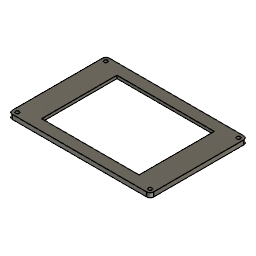
Lid V2 (Gasket) (Autodesk Fusion 360 design; units mm, degrees)
part number: 2026-01-29-14-58-12-979
Autodesk Fusion 360 part; units mm, degrees
sketch "Sketch2" plane through (0, 0, 0) normal (0, 0, 1) x (1, 0, 0)
  line L0 (-46, 50) -> (106, 50)
  line L1 (110, 46) -> (110, -56)
  line L2 (106, -60) -> (-46, -60)
  line L3 (-50, -56) -> (-50, 46)
  circle A0 centre (-45, 45) radius 2
  line L4 (30, -60) -> (30, 50) construction
  line L5 (-50, -5) -> (110, -5) construction
  arc A1 (-46, 50) -> (-50, 46) centre (-46, 46) ccw
  circle A2 centre (105, 45) radius 2
  arc A3 (110, 46) -> (106, 50) centre (106, 46) ccw
  circle A4 centre (105, -55) radius 2
  arc A5 (106, -60) -> (110, -56) centre (106, -56) ccw
  circle A6 centre (-45, -55) radius 2
  arc A7 (-50, -56) -> (-46, -60) centre (-46, -56) ccw
  point P0 (-50, 50)
  point P1 (110, 50)
  dimension "d3" = 4
  dimension "d4" = 5
  dimension "d5" = 5
  dimension "d6" = 4
  dimension "d63" = 160
  dimension "d64" = 110
  constraint horizontal L0
  constraint vertical L1
  constraint horizontal L2
  constraint vertical L3
  constraint coincident L0 L4.end
  constraint coincident L3 L5.start
  constraint coincident P0 L0
  constraint coincident P0 L3
  constraint tangent L0 A1
  constraint tangent L3 A1
  constraint symmetric P0 L4 P1
  constraint symmetric A0 L4 A2
  constraint symmetric L4 L0.start L0.end
  constraint symmetric L4 L3.end L1.start
  constraint symmetric L4 A1 A3
  constraint coincident L1 L5.end
  constraint symmetric A0 L5 A6
  constraint symmetric L5 L0.start L2.end
  constraint symmetric L5 L3.end L3.start
  constraint symmetric L5 A1 A7
  constraint symmetric L5 L1.start L1.end
  constraint symmetric L5 L0.end L2.start
  constraint symmetric L5 A2 A4
  constraint symmetric L5 A3 A5
  constraint coincident L2 L4.start
  measures "d3" diameter of A0
  measures "d4" distance of L0 A0.centre
  measures "d5" distance of L3 A0.centre
  measures "d6" radius of A1
  measures "d63" distance of L1 L3
  measures "d64" distance of L0 L2
extrude "Extrude1" add sketch "Sketch2" along normal blind 5
sketch "Sketch3" plane through (0, 0, 0) normal (0, 0, -1) x (1, 0, 0)
  circle A0 centre (105, 55) radius 2
  circle A1 centre (-45, 55) radius 2
  circle A2 centre (-45, -45) radius 2
  circle A3 centre (105, -45) radius 2
  arc A4 (-50, -46) -> (-46, -50) centre (-46, -46) ccw
  line L0 (-46, -50) -> (106, -50)
  arc A5 (106, -50) -> (110, -46) centre (106, -46) ccw
  line L1 (110, -46) -> (110, 56)
  arc A6 (110, 56) -> (106, 60) centre (106, 56) ccw
  line L2 (106, 60) -> (-46, 60)
  arc A7 (-46, 60) -> (-50, 56) centre (-46, 56) ccw
  line L3 (-50, 56) -> (-50, -46)
  line L4 (30, 60) -> (30, -50) construction
  line L5 (110, 5) -> (-50, 5) construction
  line L6 (101.7902, -41.7902) -> (-41.7901, -41.7902) construction
  line L7 (-41.7901, -41.7902) -> (-41.7901, 51.7901) construction
  line L8 (-41.7901, 51.7901) -> (101.7902, 51.7901) construction
  line L9 (101.7902, 51.7901) -> (101.7902, -41.7902) construction
  line L10 (101.7902, -41.7902) -> (-41.7901, 51.7901) construction
  line L11 (-41.7901, -41.7902) -> (101.7902, 51.7901) construction
  line L12 (95.2151, -42.8152) -> (-35.2152, -42.8152)
  line L13 (-42.8152, -35.2152) -> (-42.8152, 45.2151)
  line L14 (-35.2151, 52.8151) -> (95.2151, 52.8151)
  line L15 (102.8152, 45.2151) -> (102.8152, -35.2152)
  line L16 (88.9278, -33.6958) -> (-42.8152, 52.8151) construction
  line L17 (-37.4412, -35.28) -> (85.6746, 38.2522) construction
  line L18 (-40.7652, -35.2152) -> (-40.7652, 45.2152)
  line L19 (-35.2152, 50.7652) -> (95.2152, 50.7652)
  line L20 (100.7652, 45.2152) -> (100.7652, -35.2152)
  line L21 (98.2241, -39.1218) -> (-40.7652, 50.7652) construction
  line L22 (-34.7613, -32.5014) -> (82.9436, 35.6581) construction
  arc A8 (-35.2152, 50.7652) -> (-40.7652, 45.2152) centre (-35.2152, 45.2152) ccw
  arc A9 (-35.2151, 52.8151) -> (-42.8152, 45.2151) centre (-35.2152, 45.2151) ccw
  arc A10 (100.7652, 45.2152) -> (95.2152, 50.7652) centre (95.2152, 45.2152) ccw
  arc A11 (102.8152, 45.2151) -> (95.2151, 52.8151) centre (95.2152, 45.2151) ccw
  arc A12 (-40.7652, -35.2152) -> (-35.2152, -40.7652) centre (-35.2152, -35.2152) ccw
  arc A13 (-42.8152, -35.2152) -> (-35.2152, -42.8152) centre (-35.2152, -35.2152) ccw
  arc A14 (95.2152, -40.7652) -> (100.7652, -35.2152) centre (95.2152, -35.2152) ccw
  arc A15 (95.2151, -42.8152) -> (102.8151, -35.2152) centre (95.2151, -35.2152) ccw
  line L23 (95.2152, -40.7652) -> (-35.2152, -40.7652)
  point P0 (30, 5)
  point P1 (30, 5)
  point P2 (30, 5)
  point P3 (30, 5)
  point P4 (30, 5)
  dimension "d25" = 143.5803
  dimension "d27" = 93.5803
  dimension "d28" = 1.025
  dimension "d29" = 1.025
  dimension "d30" = 1.025
  dimension "d31" = 1.025
  dimension "d44" = 5.55
  dimension "d45" = 7.6
  constraint midpoint L2 L4.start
  constraint midpoint L0 L4.end
  constraint midpoint L1 L5.start
  constraint midpoint L3 L5.end
  constraint midpoint L4 P4
  constraint coincident P4 P3
  constraint horizontal L6
  constraint perpendicular L6 L7
  constraint parallel L6 L8
  constraint parallel L7 L9
  constraint coincident L10 P4
  constraint coincident L11 P4
  constraint horizontal L12
  constraint perpendicular L12 L13
  constraint parallel L12 L14
  constraint parallel L13 L15
  constraint coincident L16 P4
  constraint coincident L17 P4
  constraint perpendicular L18 L23
  constraint parallel L19 L23
  constraint parallel L18 L20
  constraint coincident L21 P4
  constraint coincident L22 P4
  constraint coincident L21.end L19
  constraint coincident L21.end L18
  constraint tangent L19 A8
  constraint tangent L18 A8
  constraint coincident L16.end L14
  constraint coincident L16.end L13
  constraint tangent L14 A9
  constraint tangent L13 A9
  constraint symmetric L4 L19.start L19.end
  constraint symmetric L4 L18.end L20.start
  constraint symmetric L4 A8 A10
  constraint symmetric L4 L14.start L14.end
  constraint symmetric L4 L13.end L15.start
  constraint symmetric L4 A9 A11
  constraint symmetric L5 L19.start A12.end
  constraint symmetric L5 L18.end L18.start
  constraint symmetric L5 A8 A12
  constraint symmetric L5 L14.start L12.end
  constraint symmetric L5 L13.end L13.start
  constraint symmetric L5 A9 A13
  constraint symmetric L5 L19.end A14.start
  constraint symmetric L5 L20.start L20.end
  constraint symmetric L5 A10 A14
  constraint symmetric L5 L14.end L12.start
  constraint symmetric L5 L15.start L15.end
  constraint symmetric L5 A11 A15
  measures "d25" distance of L7.end L8.end
  measures "d27" distance of L6.end L7.end
  measures "d28" distance of L9 L15
  measures "d29" distance of L8 L14
  measures "d30" distance of L8 L19
  measures "d31" distance of L9 L20
  measures "d44" radius of A8
  measures "d45" radius of A9
extrude "Extrude4" add sketch "Sketch3" along normal blind 0.8 contours L12 L13 L14 L15 A9 A11 A13 A15
draft "Draft3" angle 10 neutral plane through (0, 0, -0.8) pull (0, 0, -1) 16 faces at (8.2616, -50.7652, -0.5333) (98.4345, -49.736, -0.5333) (100.7652, -18.4051, -0.5333) (96.5236, 40.6087, -0.5333) (8.2616, 40.7652, -0.5333) (-36.2655, 40.6649, -0.5333) (-40.7652, 8.4051, -0.2667) (-39.736, -48.4345, -0.5333) (-42.8152, 8.4051, -0.5333) (-41.1892, 39.9132, -0.5333) (8.2616, 42.8152, -0.2667) (101.7969, 39.0152, -0.5333) (102.8152, -18.405, -0.5333) (97.0069, -52.6009, -0.5333) (8.2616, -52.8151, -0.2667) (-42.3972, -47.7009, -0.5333)
sketch "Sketch5" plane through (0, 0, -0.8) normal (0, 0, -1) x (1, 0, 0)
  line L0 (-35.2152, 50.7652) -> (95.2152, 50.7652)
  line L1 (100.7652, 45.2152) -> (100.7652, -35.2152)
  line L2 (95.2152, -40.7652) -> (-35.2152, -40.7652)
  line L3 (-40.7652, -35.2152) -> (-40.7652, 45.2152)
  line L4 (95.2151, 52.8151) -> (-35.2151, 52.8151)
  line L5 (-42.8152, 45.2151) -> (-42.8152, -35.2152)
  line L6 (-35.2152, -42.8152) -> (95.2151, -42.8152)
  line L7 (102.8151, -35.2152) -> (102.8152, 45.2151)
  line L8 (30, 52.8151) -> (30, -42.8152) construction
  line L9 (102.8151, 5) -> (-42.8152, 5) construction
  line L10 (101.7901, -41.7902) -> (-41.7902, -41.7902) construction
  line L11 (-41.7902, -41.7902) -> (-41.7902, 51.7901) construction
  line L12 (-41.7902, 51.7901) -> (101.7901, 51.7901) construction
  line L13 (101.7901, 51.7901) -> (101.7901, -41.7902) construction
  line L14 (101.7901, -41.7902) -> (-41.7902, 51.7901) construction
  line L15 (-41.7902, -41.7902) -> (101.7901, 51.7901) construction
  line L16 (95.2151, -42.3152) -> (-35.2151, -42.3152)
  line L17 (-42.3151, -35.2152) -> (-42.3151, 45.2151)
  line L18 (-35.2151, 52.3151) -> (95.2151, 52.3151)
  line L19 (102.3151, 45.2151) -> (102.3151, -35.2152)
  line L20 (89.0725, -33.6506) -> (-42.3151, 52.3151) construction
  line L21 (-42.3151, -42.3152) -> (89.0725, 43.6506) construction
  line L22 (95.2151, -41.2652) -> (-35.2151, -41.2652)
  line L23 (-41.2651, -35.2152) -> (-41.2651, 45.2151)
  line L24 (101.2651, 45.2151) -> (101.2651, -35.2152)
  line L25 (88.0406, -32.6798) -> (-41.2651, 51.2651) construction
  line L26 (-41.2651, -41.2652) -> (88.0406, 42.6798) construction
  arc A0 (100.7652, 45.2152) -> (95.2152, 50.7652) centre (95.2152, 45.2152) ccw
  arc A1 (95.2152, -40.7652) -> (100.7652, -35.2152) centre (95.2152, -35.2152) ccw
  arc A2 (-40.7652, -35.2152) -> (-35.2152, -40.7652) centre (-35.2152, -35.2152) ccw
  arc A3 (-35.2152, 50.7652) -> (-40.7652, 45.2152) centre (-35.2152, 45.2152) ccw
  arc A4 (-42.8152, -35.2152) -> (-35.2152, -42.8152) centre (-35.2152, -35.2152) ccw
  arc A5 (95.2151, -42.8152) -> (102.8151, -35.2152) centre (95.2152, -35.2152) ccw
  arc A6 (102.8152, 45.2151) -> (95.2151, 52.8152) centre (95.2152, 45.2152) ccw
  arc A7 (-35.2151, 52.8151) -> (-42.8151, 45.2151) centre (-35.2152, 45.2152) ccw
  arc A8 (-35.2151, 51.2651) -> (-41.2651, 45.2151) centre (-35.2151, 45.2151) ccw
  arc A9 (-35.2151, 52.3151) -> (-42.3151, 45.2151) centre (-35.2151, 45.2151) ccw
  arc A10 (101.2651, 45.2151) -> (95.2151, 51.2651) centre (95.2151, 45.2151) ccw
  arc A11 (102.3151, 45.2151) -> (95.2151, 52.3151) centre (95.2151, 45.2151) ccw
  line L27 (-35.2151, 51.2651) -> (95.2151, 51.2651)
  arc A12 (95.2151, -41.2652) -> (101.2651, -35.2152) centre (95.2151, -35.2152) ccw
  arc A13 (95.2151, -42.3152) -> (102.3151, -35.2152) centre (95.2151, -35.2152) ccw
  arc A14 (-41.2651, -35.2152) -> (-35.2151, -41.2652) centre (-35.2151, -35.2152) ccw
  arc A15 (-42.3151, -35.2152) -> (-35.2151, -42.3152) centre (-35.2151, -35.2152) ccw
  point P0 (30, 5)
  point P1 (30, 5)
  point P2 (30, 5)
  dimension "d36" = 143.5803
  dimension "d37" = 93.5803
  dimension "d38" = 0.525
  dimension "d39" = 0.525
  dimension "d40" = 0.525
  dimension "d41" = 0.525
  dimension "d50" = 6.05
  dimension "d51" = 7.1
  constraint midpoint L4 L8.start
  constraint midpoint L6 L8.end
  constraint midpoint L7 L9.start
  constraint midpoint L5 L9.end
  constraint horizontal L10
  constraint perpendicular L10 L11
  constraint parallel L10 L12
  constraint parallel L11 L13
  constraint coincident L14 P2
  constraint coincident L15 P2
  constraint midpoint L8 P2
  constraint horizontal L16
  constraint perpendicular L16 L17
  constraint parallel L16 L18
  constraint parallel L17 L19
  constraint coincident L20 P2
  constraint coincident L21 P2
  constraint coincident P2 P1
  constraint horizontal L22
  constraint perpendicular L22 L23
  constraint parallel L22 L27
  constraint parallel L23 L24
  constraint coincident L25 P2
  constraint coincident L26 P2
  constraint coincident L26.start L23
  constraint coincident L26.start L22
  constraint coincident L21.start L17
  constraint coincident L21.start L16
  constraint coincident L25.end L27
  constraint coincident L25.end L23
  constraint tangent A8 L27
  constraint tangent L23 A8
  constraint coincident L20.end L18
  constraint coincident L20.end L17
  constraint tangent L18 A9
  constraint tangent L17 A9
  constraint symmetric L8 A8.start A10.end
  constraint symmetric L8 L23.end L24.start
  constraint symmetric L8 A8 A10
  constraint symmetric L8 L18.start L18.end
  constraint symmetric L8 L17.end L19.start
  constraint symmetric L8 A9 A11
  constraint symmetric L9 A10.end L22.start
  constraint symmetric L9 L24.start L24.end
  constraint symmetric L9 A10 A12
  constraint symmetric L9 L18.end L16.start
  constraint symmetric L9 L19.start L19.end
  constraint symmetric L9 A11 A13
  constraint symmetric L9 A8.start L22.end
  constraint symmetric L9 L23.end L23.start
  constraint symmetric L9 A8 A14
  constraint symmetric L9 L18.start L16.end
  constraint symmetric L9 L17.end L17.start
  constraint symmetric L9 A9 A15
  constraint coincident L23.start A14.start
  constraint coincident L17.start A15.start
  constraint coincident L22.end A14.end
  constraint coincident L16.end A15.end
  measures "d36" distance of L11.end L12.end
  measures "d37" distance of L10.end L11.end
  measures "d38" distance of L13 L19
  measures "d39" distance of L13 L24
  measures "d40" distance of L10 L16
  measures "d41" distance of L10 L22
  measures "d50" radius of A8
  measures "d51" radius of A9
extrude "Extrude6" cut sketch "Sketch5" against normal blind 0.5 contours L16 L17 L18 L19 A9 A11 A13 A15
extrude "Extrude7" cut 1 faces at (51.7384, -20.208, 0) along direction (0, 0, 1) blind 0.5
sketch "Sketch6" plane through (0, 0, 0.5) normal (0, 0, -1) x (1, 0, 0)
  line L0 (95.2152, 50.6241) -> (-35.2152, 50.6241)
  arc A0 (-35.2152, 50.6241) -> (-40.6241, 45.2152) centre (-35.2152, 45.2152) ccw
  line L1 (-40.6241, 45.2152) -> (-40.6241, -35.2152)
  arc A1 (-40.6241, -35.2152) -> (-35.2152, -40.6241) centre (-35.2152, -35.2152) ccw
  line L2 (-35.2152, -40.6241) -> (95.2152, -40.6241)
  arc A2 (95.2152, -40.6241) -> (100.6241, -35.2152) centre (95.2152, -35.2152) ccw
  line L3 (100.6241, -35.2152) -> (100.6241, 45.2152)
  arc A3 (100.6241, 45.2152) -> (95.2152, 50.6241) centre (95.2152, 45.2152) ccw
  line L4 (30, 50.6241) -> (30, -40.6241) construction
  line L5 (-40.6241, 5) -> (100.6241, 5) construction
  line L6 (87.5, -40) -> (-27.5, -40)
  line L7 (-27.5, -40) -> (-27.5, 50)
  line L8 (-27.5, 50) -> (87.5, 50)
  line L9 (87.5, 50) -> (87.5, -40)
  line L10 (87.5, -40) -> (-27.5, 50) construction
  line L11 (-27.5, -40) -> (87.5, 50) construction
  point P0 (30, 5)
  dimension "d58" = 115
  dimension "d59" = 90
  constraint midpoint L0 L4.start
  constraint midpoint L2 L4.end
  constraint midpoint L1 L5.start
  constraint midpoint L3 L5.end
  constraint horizontal L6
  constraint perpendicular L6 L7
  constraint parallel L6 L8
  constraint parallel L7 L9
  constraint coincident L10 P0
  constraint coincident L11 P0
  constraint midpoint L5 P0
  measures "d58" distance of L7.end L8.end
  measures "d59" distance of L6.end L7.end
extrude "Extrude8" cut sketch "Sketch6" against normal blind 1.1 contours L6 L7 L8 L9
sketch "Sketch7" plane through (0, 0, 1.6) normal (0, 0, -1) x (1, 0, 0)
  line L0 (87.5, 50) -> (-27.5, 50)
  line L1 (-27.5, 50) -> (-27.5, -40)
  line L2 (-27.5, -40) -> (87.5, -40)
  line L3 (87.5, -40) -> (87.5, 50)
  line L4 (30, 50) -> (30, -40) construction
  line L5 (87.5, 5) -> (-27.5, 5) construction
  line L6 (85, -37.5) -> (-25, -37.5)
  line L7 (-25, -37.5) -> (-25, 47.5)
  line L8 (-25, 47.5) -> (85, 47.5)
  line L9 (85, 47.5) -> (85, -37.5)
  line L10 (85, -37.5) -> (-25, 47.5) construction
  line L11 (-25, -37.5) -> (85, 47.5) construction
  point P0 (30, 5)
  dimension "d62" = 110
  dimension "d65" = 85
  constraint midpoint L0 L4.start
  constraint midpoint L2 L4.end
  constraint midpoint L3 L5.start
  constraint midpoint L1 L5.end
  constraint horizontal L6
  constraint perpendicular L6 L7
  constraint parallel L6 L8
  constraint parallel L7 L9
  constraint coincident L10 P0
  constraint coincident L11 P0
  constraint midpoint L4 P0
  measures "d62" distance of L7.end L8.end
  measures "d65" distance of L6.end L7.end
extrude "Extrude9" cut sketch "Sketch7" against normal blind 8.4 contours L6 L7 L8 L9
equation "ORingDiameter = 1 mm" comment "Diamter of the O ring"
equation "ORingInnerDiameter = 150 mm" comment "Inner diamter of the o ring bore"
equation "d25 = ( ORingPerimeter - 100 mm ) / 4 + 50 mm"
equation "ORingPerimeter = 2 * 3.1412 * ( ( ORingInnerDiameter / 2 ) + ORingDiameter / 2 )"
equation "d27 = ( ORingPerimeter - 100 mm ) / 4"
equation "d28 = ( ( ORingDiameter * 1.05 ) / 2 ) + 0.5 mm"
equation "d29 = ( ( ORingDiameter * 1.05 ) / 2 ) + 0.5 mm"
equation "d30 = ( ( ORingDiameter * 1.05 ) / 2 ) + 0.5 mm"
equation "d31 = ( ( ORingDiameter * 1.05 ) / 2 ) + 0.5 mm"
equation "d32 = ORingDiameter * 0.8"
equation "d36 = ( ORingPerimeter - 100 mm ) / 4 + 50 mm"
equation "d37 = ( ORingPerimeter - 100 mm ) / 4"
equation "d38 = ( ORingDiameter * 1.05 ) / 2"
equation "d39 = ( ORingDiameter * 1.05 ) / 2"
equation "d40 = ( ORingDiameter * 1.05 ) / 2"
equation "d41 = ( ORingDiameter * 1.05 ) / 2"
equation "d44 = ( ORingDiameter ) * 6 + ORingDiameter * 0.05 - 0.5 mm"
equation "d45 = ( ORingDiameter ) * 6 + ( ORingDiameter * 1.1 ) + 0.5 mm"
equation "d50 = ( ORingDiameter ) * 6 + ORingDiameter * 0.05 - 0.0 mm"
equation "d51 = ( ORingDiameter ) * 6 + ORingDiameter * 1.1 + 0 mm"
equation "PanelWidth = 90 mm"
equation "PanelLength = 115 mm"
equation "d58 = PanelLength"
equation "d59 = PanelWidth"
equation "d62 = PanelLength - 5 mm"
equation "d65 = PanelWidth - 5 mm"
